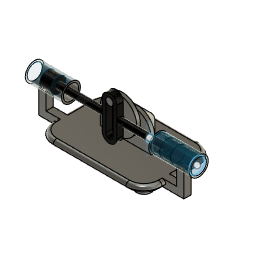
Mecanism Nebun Lab 7 (Autodesk Fusion 360 design; units mm, degrees)
Autodesk Fusion 360 part; units mm, degrees
note: some values were not read from the file. Set by a fixed rule: which sketch regions a step uses.
sketch "Sketch1" plane through (0, 0, 0) normal (0, 0, 1) x (1, 0, 0) in component "Holder"
  line L0 (-50, 50) -> (50, 50)
  line L1 (-50, -50) -> (50, -50)
  line L2 (75, -25) -> (75, 25)
  line L3 (-75, 25) -> (-75, -25)
  circle A0 centre (-50, -25) radius 25
  circle A1 centre (50, -25) radius 25
  circle A2 centre (50, 25) radius 25
  circle A3 centre (-50, 25) radius 25
  line L4 (-35, 25) -> (35, 25)
  line L5 (35, 25) -> (35, 0)
  line L6 (35, 0) -> (-35, 0)
  line L7 (-35, 0) -> (-35, 25)
  circle A4 centre (50, 25) radius 10
  circle A5 centre (50, -25) radius 10
  circle A6 centre (-50, -25) radius 10
  circle A7 centre (-50, 25) radius 10
  line L8 (100, -10) -> (90, -10)
  line L9 (90, -10) -> (90, -20)
  line L10 (90, -20) -> (100, -20)
  line L11 (100, -20) -> (100, -10)
  line L12 (-100, -10) -> (-90, -10)
  line L13 (-90, -10) -> (-90, -20)
  line L14 (-90, -20) -> (-100, -20)
  line L15 (-100, -20) -> (-100, -10)
  constraint horizontal L0
  constraint horizontal L1
  constraint perpendicular L1 L2
  constraint perpendicular L1 L3
  constraint coincident L3.end A0
  constraint coincident L1.end A1
  constraint coincident L0.end A2
  constraint tangent L0 A2
  constraint coincident L0.start A3
  constraint tangent L0 A3
  constraint horizontal L4
  constraint vertical L5
  constraint horizontal L6
  constraint vertical L7
  constraint concentric A2 A4
  constraint concentric A1 A5
  constraint concentric A0 A6
  constraint concentric A3 A7
  constraint horizontal L8
  constraint vertical L9
  constraint horizontal L10
  constraint vertical L11
  constraint horizontal L12
  constraint vertical L13
  constraint horizontal L14
  constraint vertical L15
extrude "Extrude1" add sketch "Sketch1" along normal blind 20 and the other way blind -10 contours L0 A2 A3 L4 | A3 L4 L7 | A2 L4 L5 | A2 A3 L4 L5 L6 L7 | A3 L4 L7 | L3 A0 A3 | L2 A1 A2 | A2 L4 L5 | L1 A0 A1 A2 A3 L5 L6 L7 | A0 | A1 | A4 | A5 | A6 | A7 makes body 1 in component "Holder"
extrude "Extrude2" add sketch "Sketch1" along normal blind 20 contours A4 | A5 | A6 | A7 bodies 1 in component "Holder"
extrude "Extrude3" add sketch "Sketch1" along normal blind 65 and the other way blind -20 contours A2 A3 L4 L5 L6 L7 | A3 L4 L7 | A2 L4 L5 picked at (-28.4063, 23.8993) picked at (28.4063, 23.8993) bodies 1 in component "Holder"
fillet "Fillet1" radius 25 1 edges at (35, 12.5, 65) on bodies 1 in component "Holder"
fillet "Fillet2" radius 25 1 edges at (-35, 12.5, 65) on bodies 1 in component "Holder"
sketch "Sketch2" plane through (0, 0, 0) normal (0, -1, 0) x (1, 0, 0) in component "Holder"
  arc A0 (-10, 65) -> (-35, 40) centre (-10, 40) ccw
  line L0 (-35, 40) -> (-35, 20)
  line L1 (35, 20) -> (35, 40)
  arc A1 (35, 40) -> (10, 65) centre (10, 40) ccw
  line L2 (10, 65) -> (-10, 65)
  circle A2 centre (0, 55) radius 7.5
  line L3 (-35, 20) -> (35, 20)
  dimension "d15" = 15
  measures "d15" diameter of A2
extrude "Extrude4" add sketch "Sketch2" along normal blind 15 contours A2 bodies 1 in component "Holder"
sketch "Sketch1 (2)" plane through (0, 0, 0) normal (0, 1, 0) x (1, 0, 0) in component "Wheel"
  circle A0 centre (0, -55) radius 7.5
  circle A1 centre (0, -55) radius 25
  circle A2 centre (0, -75) radius 5
  dimension "d18" = 15
  dimension "d19" = 50
  constraint concentric A0 A1
  measures "d18" diameter of A0
  measures "d19" diameter of A1
extrude "Extrude1'" add sketch "Sketch1 (2)" along normal blind -5 and the other way blind 10 separate body contours A2 | A1 makes body 2 in component "Wheel"
extrude "Extrude2'" add sketch "Sketch1 (2)" along normal blind -10 and the other way blind 20 contours A2 bodies 2 in component "Wheel"
sketch "Sketch1 (3)" plane through (0, 0, 0) normal (0, 1, 0) x (1, 0, 0) in component "Piston"
  line L0 (-5, -75) -> (-5, -35)
  line L1 (5, -75) -> (5, -35)
  circle A0 centre (0, -75) radius 5
  circle A1 centre (0, -35) radius 5
  circle A2 centre (0, -75) radius 10
  circle A3 centre (0, -35) radius 10
  line L2 (10, -75) -> (10, -35)
  line L3 (-10, -75) -> (-10, -35)
  constraint vertical L0
  constraint parallel L0 L1
  constraint coincident L0.start A0
  constraint tangent L0 A0
  constraint coincident L1.start A0
  constraint coincident L0.end A1
  constraint tangent L0 A1
  constraint coincident L1.end A1
  constraint coincident A2 L2.start
  constraint coincident A3 L2.end
  constraint tangent A3 L2
  constraint parallel L1 L2
  constraint coincident A2 L3.start
  constraint coincident A3 L3.end
  constraint tangent A3 L3
  constraint parallel L0 L3
extrude "Extrude1''" add sketch "Sketch1 (3)" along normal blind -20 and the other way blind 11 separate body contours L0 L1 A0 A2 | L0 A2 A3 L3 | L0 L1 A1 A3 | L1 A2 A3 L2 picked at (8.2775, -75.7452) picked at (8.2961, -35.4968) makes body 3 in component "Piston"
sketch "Sketch2 (2)" plane through (10, 0, 0) normal (1, 0, 0) x (0, 1, 0) in component "Piston"
  line L0 (-11, 35) -> (-11, 75)
  line L1 (-11, 75) -> (-20, 75)
  line L2 (-20, 75) -> (-20, 35)
  line L3 (-20, 35) -> (-11, 35)
  circle A0 centre (-15.5, 55) radius 4.5
  constraint tangent L2 A0
extrude "Extrude2''" add sketch "Sketch2 (2)" along normal blind 65 contours A0 bodies 3 in component "Piston"
extrude "Extrude3'" add sketch "Sketch2 (2)" along normal blind -20 and the other way blind 85 contours A0 bodies 3 in component "Piston"
extrude "Extrude5" cut 1 faces at (-0.1993, -15, 57.3272) along direction (0, 1, 0) blind 5 on bodies 1 bodies 1 in component "Holder"
sketch "Sketch3" plane through (75, 0, 0) normal (1, 0, 0) x (0, 1, 0) in component "Piston"
  circle A0 centre (-15.5, 55) radius 4.5
  circle A1 centre (-15.5, 55) radius 10.5
  constraint concentric A0 A1
extrude "Extrude4'" add sketch "Sketch3" 1 faces at (75, -14.3041, 52.9823) along normal blind 15 on bodies 3 bodies 3 in component "Piston"
extrude "Extrude5'" add sketch "Sketch3" along normal blind -165 and the other way blind 150 contours A0 | A1 bodies 3 in component "Piston"
sketch "Sketch3 (2)" plane through (75, 0, 0) normal (1, 0, 0) x (0, 1, 0) in component "Holder"
  line L0 (-25, 10) -> (25, 10)
  line L1 (25, 10) -> (25, 20)
  line L2 (25, 20) -> (-25, 20)
  line L3 (-25, 20) -> (-25, 10)
  line L4 (-20, 20) -> (-10, 20)
  line L5 (-10, 20) -> (-10, 10)
  line L6 (-10, 10) -> (-20, 10)
  line L7 (-20, 10) -> (-20, 20)
  constraint horizontal L4
  constraint vertical L5
  constraint horizontal L6
  constraint vertical L7
  constraint coincident L0 L5.end
extrude "Extrude6" add sketch "Sketch3 (2)" along normal blind 25 contours L0 L2 L4 L5 L6 L7 bodies 1 in component "Holder"
extrude "Extrude7" add sketch "Sketch1" along normal blind 44 and the other way blind -20 contours L8 L9 L10 L11 bodies 1 in component "Holder"
ref_plane "WorkPlane1" through (75, 0, 0) normal (1, 0, 0) x (0, 1, 0) in component "Holder"
ref_plane "WorkPlane2" through (75, 0, 0) normal (1, 0, 0) x (0, 1, 0) in component "Holder"
ref_plane "WorkPlane3" through (75, 0, 0) normal (1, 0, 0) x (0, 1, 0) in component "Holder"
ref_plane "WorkPlane4" through (75, -15.5, 55) normal (1, 0, 0) x (0, 1, 0) in component "Holder"
sketch "Sketch5" plane through (75, -15.5, 55) normal (1, 0, 0) x (0, 1, 0) in component "Holder"
  circle A0 centre (0, 0) radius 10.5
  circle A1 centre (0, 0) radius 13
  dimension "d60" = 21
  constraint concentric A0 A1
  measures "d60" diameter of A0
extrude "Extrude8" add sketch "Sketch5" along normal blind 41 separate body makes body 4 in component "Holder"
move_body "Move1" bodies 3 to x (1, 0, 0) y (0, 1, 0) z (0, 0, 1) at (-41, 0, 0) in component "Piston"
extrude "Extrude9" add sketch "Sketch5" against normal blind 15 bodies 4 in component "Holder"
extrude "Extrude10" add sketch "Sketch3 (2)" against normal blind 175 contours L0 L2 L4 L5 L6 L7 bodies 1 in component "Holder"
extrude "Extrude11" add sketch "Sketch1" along normal blind 20 and the other way blind -43 contours L12 L13 L14 L15 bodies 1 in component "Holder"
extrude "Extrude12" add sketch "Sketch5" along normal blind -185 and the other way blind 135 bodies 1 4 in component "Holder"
chamfer "Chamfer1" distance 20 angle 45 5 edges at (0, 25, 65) (-27.6777, 25, 57.6777) (-35, 25, 30) (35, 25, 30) (27.6777, 25, 57.6777) on bodies 1 in component "Holder"
fillet "Fillet3" radius 5 10 edges at (75, 7.5, 20) (67.6777, 42.6777, 20) (0, 50, 20) (-67.6777, 42.6777, 20) (-75, 7.5, 20) (-75, -22.5, 20) (-67.6777, -42.6777, 20) (0, -50, 20) (67.6777, -42.6777, 20) (75, -22.5, 20) on bodies 1 in component "Holder"
chamfer "Chamfer2" distance 5 angle 45 10 edges at (67.6777, -42.6777, 10) (75, -22.5, 10) (-75, -22.5, 10) (-67.6777, -42.6777, 10) (0, -50, 10) (67.6777, 42.6777, 10) (0, 50, 10) (-67.6777, 42.6777, 10) (-75, 7.5, 10) (75, 7.5, 10) on bodies 1 in component "Holder"
component "Piston" placed x (1, 0, 0) y (0, 1, 0) z (0, 0, 1) at (41, 0, 0)
component "Wheel" placed x (1, 0, 0) y (0, 1, 0) z (0, 0, 1) at (0, 0, 0)
component "Holder" placed x (1, 0, 0) y (0, 1, 0) z (0, 0, 1) at (0, 0, 0)
